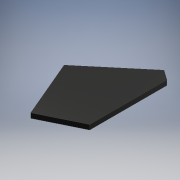
# Autodesk Inventor part: Tafe WA LOGO backplate
Saved by Autodesk Inventor 2018 (Build 220112000, 112)
## iProperties
Created: 2018-10-30
Part Number: Tafe WA LOGO backplate
Material: Generic
Document SubType Name: Modeling
Designer: Otis PC
Density: 1 g/cm^3
Appearance: Glossy - Black
Author: Otis PC
Autodesk Inventor part; units mm, degrees
ref_plane "YZ Plane" through (0, 0, 0) normal (1, 0, 0) x (0, 1, 0)
ref_plane "XZ Plane" through (0, 0, 0) normal (0, 1, 0) x (-1, 0, 0)
ref_plane "XY Plane" through (0, 0, 0) normal (0, 0, 1) x (1, 0, 0)
sketch "Sketch1" plane through (0, 0, 0) normal (0, 0, 1) x (1, 0, 0)
  line L0 (18.5838, -6.189) -> (18.5838, 42.8381)
  line L1 (18.5838, 42.8381) -> (12.2763, 47.2547)
  line L2 (12.2763, 47.2547) -> (-22.1957, 18.3292)
  line L3 (-22.1957, 18.3292) -> (-6.5665, -18.491)
  line L4 (18.5838, -6.189) -> (-6.5665, -18.491)
  point P0 (0, 0)
  point P1 (0, 0)
  dimension "d0" = 125
  dimension "d1" = 116.065
  dimension "d2" = 50
  dimension "d3" = 23
  dimension "d4" = 18.5838
  dimension "d5" = 45.7502
  dimension "d6" = 13.7251
  dimension "d7" = 28.3081
  dimension "d8" = 13.2695
  constraints: 10 end point, 1 vertical
  measures "d0" angle of L1 L0
  measures "d1" angle of L0 L4
  measures "d2" angle of L0 L2
  measures "d3" angle of L0 L3
  measures "d4" distance from line of point (0, 0) L0
  measures "d5" distance from line of point (0, 0) L1
  measures "d6" distance from line of point (0, 0) L4
  measures "d7" distance from line of point (0, 0) L2
  measures "d8" distance from line of point (0, 0) L3
extrude "Extrusion1" add sketch "Sketch1" against normal blind 3
body "Solid1"
